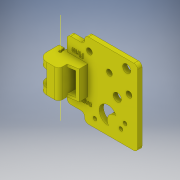
# Autodesk Inventor part: Catch
Saved by Autodesk Inventor 2016 (Build 200138000, 138)
## iProperties
Created: 2016-11-16
Part Number: Catch
Material: ABS Plastic
Document SubType Name: Modeling
Designer: brownadam
Density: 1.06 g/cm^3
Appearance: Yellow
Author: brownadam
Autodesk Inventor part; units mm, degrees
note: some values were not read from the file. Chosen so that the rebuilt part matches the saved one: direction of "Emboss1".
ref_plane "YZ Plane" through (0, 0, 0) normal (1, 0, 0) x (0, 1, 0)
ref_plane "XZ Plane" through (0, 0, 0) normal (0, 1, 0) x (-1, 0, 0)
ref_plane "XY Plane" through (0, 0, 0) normal (0, 0, 1) x (1, 0, 0)
sketch "Sketch1" plane through (0, 0, 0) normal (0, 0, 1) x (1, 0, 0)
  line L0 (30.48, 0) -> (30.48, 14.732)
  line L1 (28.8925, 16.3195) -> (9.2075, 16.3195)
  line L2 (0, 11.176) -> (0, 3.429)
  line L3 (7.62, 14.732) -> (7.62, 14.351)
  line L4 (6.0325, 12.7635) -> (1.5875, 12.7635)
  line L5 (7.62, 0) -> (30.48, 0) construction
  arc A0 (1.5875, 12.7635) -> (0, 11.176) centre (1.5875, 11.176) ccw
  arc A1 (6.0325, 12.7635) -> (7.62, 14.351) centre (6.0325, 14.351) ccw
  arc A2 (9.2075, 16.3195) -> (7.62, 14.732) centre (9.2075, 14.732) ccw
  arc A3 (30.48, 14.732) -> (28.8925, 16.3195) centre (28.8925, 14.732) ccw
  line L6 (0, 3.429) -> (2.2606, 3.429)
  line L7 (2.2606, 3.429) -> (2.2606, 0)
  line L8 (30.48, 0) -> (2.2606, 0) construction
  line L9 (30.48, 0) -> (30.48, -14.732)
  line L10 (28.8925, -16.3195) -> (9.2075, -16.3195)
  line L11 (0, -11.176) -> (0, -3.429)
  line L12 (6.0325, -12.7635) -> (1.5875, -12.7635)
  arc A4 (0, -11.176) -> (1.5875, -12.7635) centre (1.5875, -11.176) ccw
  arc A5 (7.62, -14.351) -> (6.0325, -12.7635) centre (6.0325, -14.351) ccw
  arc A6 (7.62, -14.732) -> (9.2075, -16.3195) centre (9.2075, -14.732) ccw
  arc A7 (28.8925, -16.3195) -> (30.48, -14.732) centre (28.8925, -14.732) ccw
  line L13 (0, -3.429) -> (2.2606, -3.429)
  line L14 (2.2606, -3.429) -> (2.2606, 0)
  line L15 (7.62, -14.732) -> (7.62, -14.351)
  point P0 (0, 0)
  dimension "d4" = 30.48
  dimension "d5" = 7.62
  dimension "d6" = 3.556
  dimension "d8" = 1.5875
  dimension "d9" = 1.5875
  dimension "d10" = 1.5875
  dimension "d11" = 1.5875
  dimension "d13" = 16.3195
  dimension "d14" = 2.2606
  dimension "d16" = 3.429
  constraints: 32 end point, 16 point on circle, 14 symmetric about line, 8 centre point, 8 tangent, 2 horizontal alignment, 2 perpendicular, 1 collinear, 1 horizontal, 1 parallel, 1 point on line, 1 vertical, 1 vertical alignment, 4 other
  measures "d4" distance between parallel lines of L0 L2
  measures "d5" distance between parallel lines of L3 L2
  measures "d6" distance between parallel lines of L4 L1
  measures "d8" radius of A0
  measures "d9" radius of A1
  measures "d10" radius of A2
  measures "d11" radius of A3
  measures "d13" distance between parallel lines of L5 L1
  measures "d14" distance of L2.end L6.end
  measures "d16" distance from line of L7.end L6
extrude "Extrusion1" add sketch "Sketch1" against normal blind 1.905
sketch "Sketch2" plane through (0, 0, 0) normal (0, 0, 1) x (1, 0, 0)
  line L0 (30.48, 14.732) -> (30.48, -14.732) projected
  line L1 (9.2075, 16.3195) -> (28.8925, 16.3195) projected
  line L2 (-4.318, 6.1595) -> (9.017, 6.1595)
  line L3 (9.017, 6.1595) -> (9.017, -6.1595)
  line L4 (9.017, -6.1595) -> (-4.318, -6.1595)
  line L5 (-4.318, -6.1595) -> (-4.318, 6.1595)
  point P0 (0, 0)
  dimension "d19" = 13.335
  dimension "d20" = 12.319
  dimension "d21" = 10.16
  dimension "d22" = 21.463
  constraints: 8 end point, 2 parallel, 1 horizontal, 1 perpendicular
  measures "d19" distance of L2.start L2.end
  measures "d20" distance of L2.end L3.end
  measures "d21" distance between parallel lines of L1 L2
  measures "d22" distance between parallel lines of L0 L3
extrude "Extrusion2" add sketch "Sketch2" along normal blind 8.255
sketch "Sketch3" plane through (0, 0, 8.255) normal (0, 0, 1) x (1, 0, 0)
  line L0 (9.017, 6.1595) -> (-4.318, 6.1595) projected
  line L1 (-4.318, 6.1595) -> (-4.318, -6.1595) projected
  line L2 (-4.318, -6.1595) -> (9.017, -6.1595) projected
  line L3 (9.017, -6.1595) -> (9.017, 6.1595) projected
  line L4 (-4.318, 3.429) -> (-0.508, 3.429)
  line L5 (-0.508, 3.429) -> (-0.508, -3.429)
  line L6 (-0.508, -3.429) -> (-4.318, -3.429)
  line L7 (-4.318, -3.429) -> (-4.318, 3.429)
  line L8 (9.017, 5.0165) -> (4.572, 5.0165)
  line L9 (4.572, 5.0165) -> (4.572, -5.0165)
  line L10 (4.572, -5.0165) -> (9.017, -5.0165)
  line L11 (9.017, -5.0165) -> (9.017, 5.0165)
  line L12 (4.572, 5.0165) -> (7.747, 5.0165)
  line L13 (7.747, 5.0165) -> (7.747, -5.0165)
  line L14 (7.747, -5.0165) -> (4.572, -5.0165)
  line L15 (4.572, -5.0165) -> (4.572, 5.0165)
  line L16 (4.572, 5.0165) -> (4.572, 6.1595)
  line L17 (4.572, -5.0165) -> (4.572, -6.1595)
  point P0 (0, 0)
  dimension "d25" = 3.81
  dimension "d27" = 2.7305
  dimension "d28" = 5.08
  dimension "d29" = 1.143
  dimension "d30" = 1.143
  dimension "d31" = 1.27
  dimension "d38" = 2.7305
  constraints: 28 end point, 6 parallel, 6 point on line, 4 perpendicular, 3 horizontal
  measures "d25" distance of L5.end L6.end
  measures "d27" distance between parallel lines of L0 L4
  measures "d28" distance between parallel lines of L9 L5
  measures "d29" distance between parallel lines of L2 L10
  measures "d30" distance between parallel lines of L0 L8
  measures "d31" distance between parallel lines of L13 L11
  measures "d38" distance between parallel lines of L6 L2
extrude "Extrusion3" cut sketch "Sketch3" against normal through all contours L4 L5 L6 L1
extrude "Extrusion4" cut sketch "Sketch3" against normal up to surface (8.255 mm away) contours L8 L13 L10 L9
sketch "Sketch4" plane through (0, 0, 0) normal (0, 0, -1) x (-1, 0, 0)
  line L0 (0.508, 3.429) -> (0, 3.429)
  line L1 (0, 3.429) -> (0, 6.1595)
  line L2 (0, 6.1595) -> (0.508, 6.1595)
  line L3 (0.508, 6.1595) -> (0.508, 3.429)
  line L4 (0.508, -3.429) -> (0, -3.429)
  line L5 (0, -3.429) -> (0, -6.1595)
  line L6 (0, -6.1595) -> (0.508, -6.1595)
  line L7 (0.508, -6.1595) -> (0.508, -3.429)
  line L8 (4.318, -3.429) -> (0.508, -3.429) projected
  line L9 (0.508, -3.429) -> (0.508, 3.429) projected
  line L10 (0.508, 3.429) -> (4.318, 3.429) projected
  line L11 (4.318, 3.429) -> (4.318, 6.1595) projected
  line L12 (4.318, 6.1595) -> (0, 6.1595) projected
  line L13 (0, 3.429) -> (0, 6.1595) projected
  line L14 (-2.2606, 3.429) -> (0, 3.429) projected
  line L15 (-2.2606, -3.429) -> (-2.2606, 3.429) projected
  line L16 (0, -3.429) -> (-2.2606, -3.429) projected
  line L17 (0, -6.1595) -> (0, -3.429) projected
  line L18 (0, -6.1595) -> (4.318, -6.1595) projected
  line L19 (4.318, -6.1595) -> (4.318, -3.429) projected
  line L20 (4.318, 6.1595) -> (0.508, 6.1595)
  line L21 (0.508, 6.1595) -> (0.508, 3.429)
  line L22 (0.508, 3.429) -> (4.318, 3.429)
  line L23 (4.318, 3.429) -> (4.318, 6.1595)
  line L24 (0.508, -3.429) -> (4.318, -3.429) projected
  line L25 (4.318, -3.429) -> (0.508, -3.429)
  line L26 (0.508, -3.429) -> (0.508, -6.1595)
  line L27 (0.508, -6.1595) -> (4.318, -6.1595)
  line L28 (4.318, -6.1595) -> (4.318, -3.429)
  point P0 (0, 0)
  constraints: 32 end point, 8 parallel, 4 horizontal, 4 perpendicular
extrude "Extrusion5" add sketch "Sketch4" along normal up to surface (1.905 mm away) contours L0 L1 L2 L3 | L7 L6 L5 L4
extrude "Extrusion6" add sketch "Sketch4" along normal blind 0.889 contours L3 L12 L11 L10 | L8 L19 L18 L7
sketch "Sketch6" plane through (0, -6.1595, 0) normal (0, -1, 0) x (1, 0, 0)
  line L0 (-4.318, 8.255) -> (9.017, 8.255) projected
  line L1 (-4.318, 8.255) -> (-4.318, -0.889) projected
  line L2 (-0.508, -0.889) -> (-4.318, -0.889) projected
  line L3 (9.017, 0) -> (9.017, 3.81)
  line L4 (9.017, 0) -> (9.017, 8.255) projected
  line L5 (7.747, 8.255) -> (4.572, 8.255) construction
  line L6 (4.572, 8.255) -> (4.572, 0) construction
  line L7 (4.572, 8.255) -> (4.572, 0) construction
  line L8 (9.017, 3.81) -> (4.572, 4.572)
  line L9 (4.572, 8.255) -> (4.572, 0) projected
  line L10 (4.572, 4.572) -> (4.572, 8.255)
  line L11 (4.572, 8.255) -> (-4.318, 8.255)
  line L12 (-4.318, -0.889) -> (-4.318, 8.255) projected
  line L13 (-4.318, 8.255) -> (-4.318, -0.889)
  line L14 (-4.318, -0.889) -> (-2.032, -0.889)
  line L15 (-2.032, -0.889) -> (-1.905, 0.8471)
  line L16 (-0.508, -0.889) -> (-0.508, -1.905) projected
  line L17 (-0.508, -0.889) -> (-1.143, -0.889)
  line L18 (-1.143, -0.889) -> (-1.27, 0.8471)
  line L19 (-1.905, 0.8471) -> (-1.27, 0.8471) construction
  arc A0 (-1.27, 0.8471) -> (-1.905, 0.8471) centre (-1.5875, 1.3284) ccw
  line L20 (4.572, 8.255) -> (9.017, 8.255)
  line L21 (9.017, 8.255) -> (9.017, 3.81)
  point P0 (-1.5875, 0.8471)
  point P1 (-1.5875, 1.905)
  dimension "d41" = 3.81
  dimension "d42" = 3.683
  dimension "d43" = 2.286
  dimension "d44" = 0.635
  dimension "d45" = 1.1532
  dimension "d46" = 0.635
  dimension "d47" = 6.35
  dimension "d48" = 1.7361
  constraints: 26 end point, 5 collinear, 4 point on line, 3 point on circle, 2 horizontal, 1 centre point, 1 coincident, 1 equal length, 1 midpoint, 1 vertical alignment
  measures "d41" distance of L3.start L3.end
  measures "d42" distance of L5.end L8.end
  measures "d43" distance of L1.end L14.end
  measures "d44" distance of L2.start L17.end
  measures "d45" diameter of A0
  measures "d46" distance of L18.end L15.end
  measures "d47" distance from line of point (-1.588, 1.905) L11
  measures "d48" vertical distance of L14.end L15.end
extrude "Extrusion7" cut sketch "Sketch6" against normal through all
fillet "Fillet1" radius 1.5875 1 edges at (4.572, 0, 8.255)
fillet "Fillet2" radius 3.81 2 edges at (-4.318, -4.7942, 8.255) (-4.318, 4.7943, 8.255)
sketch "Sketch7" plane through (0, 0, 0) normal (0, 0, 1) x (1, 0, 0)
  arc A0 (21.1133, -7.0794) -> (17.8739, -12.4712) centre (17.6502, -8.6677) ccw
  arc A1 (21.1133, -7.0794) -> (17.8739, -12.4712) centre (20.916, -10.6299) ccw
  line L0 (7.3431, 7.1617) -> (-0.2045, 7.1617) construction
  line L1 (-0.2045, 7.1617) -> (-0.2045, 10.7769) construction
  line L2 (-0.2045, 10.7769) -> (7.3431, 10.7769) construction
  line L3 (7.3431, 10.7769) -> (7.3431, 7.1617) construction
  line L4 (0.5888, -7.1353) -> (10.8131, -7.1353) construction
  line L5 (10.8131, -7.1353) -> (10.8131, -9.1082) construction
  line L6 (10.8131, -9.1082) -> (0.5888, -9.1082) construction
  line L7 (0.5888, -9.1082) -> (0.5888, -7.1353) construction
  spline S0 degree 2 poles (1.3128, -9.1082) (1.106, -9.1082) (0.8157, -9.0218) (0.6876, -8.96) knots 0 0 0 1 2 2 2
  line L8 (0.6876, -8.96) -> (0.6876, -8.642)
  line L9 (0.6876, -8.642) -> (0.7061, -8.642)
  spline S1 degree 2 poles (0.7061, -8.642) (0.8312, -8.7594) (1.1477, -8.889) (1.2943, -8.889) knots 0 0 0 1 2 2 2
  spline S2 degree 2 poles (1.2943, -8.889) (1.5043, -8.889) (1.7188, -8.7146) (1.7188, -8.571) knots 0 0 0 1 2 2 2
  spline S3 degree 2 poles (1.7188, -8.571) (1.7188, -8.4568) (1.6062, -8.3148) (1.4842, -8.2792) knots 0 0 0 1 2 2 2
  spline S4 degree 2 poles (1.4842, -8.2792) (1.3962, -8.2545) (1.2495, -8.2206) (1.1399, -8.1928) knots 0 0 0 1 2 2 2
  spline S5 degree 2 poles (1.1399, -8.1928) (1.0411, -8.1665) (0.8852, -8.0878) (0.825, -8.0245) knots 0 0 0 1 2 2 2
  spline S6 degree 2 poles (0.825, -8.0245) (0.7663, -7.9612) (0.7015, -7.7914) (0.7015, -7.6803) knots 0 0 0 1 2 2 2
  spline S7 degree 2 poles (0.7015, -7.6803) (0.7015, -7.4487) (1.0627, -7.1353) (1.3422, -7.1353) knots 0 0 0 1 2 2 2
  spline S8 degree 2 poles (1.3422, -7.1353) (1.5027, -7.1353) (1.7868, -7.1986) (1.9087, -7.2588) knots 0 0 0 1 2 2 2
  line L10 (1.9087, -7.2588) -> (1.9087, -7.5614)
  line L11 (1.9087, -7.5614) -> (1.8902, -7.5614)
  spline S9 degree 2 poles (1.8902, -7.5614) (1.7991, -7.478) (1.5151, -7.3545) (1.3591, -7.3545) knots 0 0 0 1 2 2 2
  spline S10 degree 2 poles (1.3591, -7.3545) (1.1832, -7.3545) (0.9655, -7.5197) (0.9655, -7.654) knots 0 0 0 1 2 2 2
  spline S11 degree 2 poles (0.9655, -7.654) (0.9655, -7.7744) (1.0936, -7.918) (1.214, -7.9504) knots 0 0 0 1 2 2 2
  spline S12 degree 2 poles (1.214, -7.9504) (1.2943, -7.972) (1.5274, -8.0276) (1.6046, -8.0508) knots 0 0 0 1 2 2 2
  spline S13 degree 2 poles (1.6046, -8.0508) (1.8007, -8.111) (1.9828, -8.3533) (1.9828, -8.5309) knots 0 0 0 1 2 2 2
  spline S14 degree 2 poles (1.9828, -8.5309) (1.9828, -8.6436) (1.8917, -8.8597) (1.8099, -8.9353) knots 0 0 0 1 2 2 2
  spline S15 degree 2 poles (1.8099, -8.9353) (1.7188, -9.0187) (1.4873, -9.1082) (1.3128, -9.1082) knots 0 0 0 1 2 2 2
  spline S16 degree 2 poles (2.8427, -9.1067) (2.5, -9.1067) (2.1233, -8.7223) (2.1233, -8.3672) knots 0 0 0 1 2 2 2
  spline S17 degree 2 poles (2.1233, -8.3672) (2.1233, -8.0183) (2.4892, -7.6046) (2.784, -7.6046) knots 0 0 0 1 2 2 2
  spline S18 degree 2 poles (2.784, -7.6046) (2.9168, -7.6046) (3.1221, -7.6818) (3.1978, -7.7636) knots 0 0 0 1 2 2 2
  spline S19 degree 2 poles (3.1978, -7.7636) (3.275, -7.8454) (3.3568, -8.0816) (3.3568, -8.253) knots 0 0 0 1 2 2 2
  line L12 (3.3568, -8.253) -> (3.3568, -8.3842)
  line L13 (3.3568, -8.3842) -> (2.3672, -8.3842)
  spline S20 degree 2 poles (2.3672, -8.3842) (2.3672, -8.6328) (2.6173, -8.8967) (2.8396, -8.8967) knots 0 0 0 1 2 2 2
  spline S21 degree 2 poles (2.8396, -8.8967) (2.9183, -8.8967) (3.0712, -8.8612) (3.1329, -8.8335) knots 0 0 0 1 2 2 2
  spline S22 degree 2 poles (3.1329, -8.8335) (3.1978, -8.8026) (3.2873, -8.7485) (3.3166, -8.7238) knots 0 0 0 1 2 2 2
  line L14 (3.3166, -8.7238) -> (3.3305, -8.7238)
  line L15 (3.3305, -8.7238) -> (3.3305, -8.9863)
  spline S23 degree 2 poles (3.3305, -8.9863) (3.2888, -9.0033) (3.1623, -9.0527) (3.1129, -9.0666) knots 0 0 0 1 2 2 2
  spline S24 degree 2 poles (3.1129, -9.0666) (3.0434, -9.0866) (2.9292, -9.1067) (2.8427, -9.1067) knots 0 0 0 1 2 2 2
  spline S25 degree 2 poles (3.1221, -8.2005) (3.119, -8.1033) (3.0789, -7.9612) (3.0403, -7.9134) knots 0 0 0 1 2 2 2
  spline S26 degree 2 poles (3.0403, -7.9134) (2.9986, -7.8593) (2.8674, -7.8022) (2.7701, -7.8022) knots 0 0 0 1 2 2 2
  spline S27 degree 2 poles (2.7701, -7.8022) (2.6744, -7.8022) (2.5401, -7.8593) (2.4846, -7.9149) knots 0 0 0 1 2 2 2
  spline S28 degree 2 poles (2.4846, -7.9149) (2.4305, -7.972) (2.3749, -8.1094) (2.3672, -8.2005) knots 0 0 0 1 2 2 2
  line L16 (2.3672, -8.2005) -> (3.1221, -8.2005)
  line L17 (4.723, -9.0743) -> (4.4822, -9.0743)
  line L18 (4.4822, -9.0743) -> (4.4822, -8.2592)
  spline S29 degree 2 poles (4.4822, -8.2592) (4.4822, -8.1604) (4.4637, -7.9906) (4.4359, -7.9396) knots 0 0 0 1 2 2 2
  spline S30 degree 2 poles (4.4359, -7.9396) (4.4065, -7.8856) (4.3016, -7.8331) (4.212, -7.8331) knots 0 0 0 1 2 2 2
  spline S31 degree 2 poles (4.212, -7.8331) (4.1225, -7.8331) (3.9326, -7.9288) (3.8415, -8.006) knots 0 0 0 1 2 2 2
  line L19 (3.8415, -8.006) -> (3.8415, -9.0743)
  line L20 (3.8415, -9.0743) -> (3.6007, -9.0743)
  line L21 (3.6007, -9.0743) -> (3.6007, -7.6448)
  line L22 (3.6007, -7.6448) -> (3.8415, -7.6448)
  line L23 (3.8415, -7.6448) -> (3.8415, -7.8038)
  spline S32 degree 2 poles (3.8415, -7.8038) (3.9496, -7.7065) (4.158, -7.6046) (4.2753, -7.6046) knots 0 0 0 1 2 2 2
  spline S33 degree 2 poles (4.2753, -7.6046) (4.4853, -7.6046) (4.723, -7.8825) (4.723, -8.1465) knots 0 0 0 1 2 2 2
  line L24 (4.723, -8.1465) -> (4.723, -9.0743)
  spline S34 degree 2 poles (5.447, -9.1082) (5.3035, -9.1082) (5.0549, -9.0311) (4.9731, -8.9878) knots 0 0 0 1 2 2 2
  line L25 (4.9731, -8.9878) -> (4.9731, -8.7177)
  line L26 (4.9731, -8.7177) -> (4.9854, -8.7177)
  spline S35 degree 2 poles (4.9854, -8.7177) (5.0163, -8.7424) (5.0997, -8.801) (5.1691, -8.8335) knots 0 0 0 1 2 2 2
  spline S36 degree 2 poles (5.1691, -8.8335) (5.2294, -8.8628) (5.3776, -8.906) (5.4563, -8.906) knots 0 0 0 1 2 2 2
  spline S37 degree 2 poles (5.4563, -8.906) (5.5134, -8.906) (5.6446, -8.8798) (5.6755, -8.8582) knots 0 0 0 1 2 2 2
  spline S38 degree 2 poles (5.6755, -8.8582) (5.7203, -8.8288) (5.7604, -8.7624) (5.7604, -8.6945) knots 0 0 0 1 2 2 2
  spline S39 degree 2 poles (5.7604, -8.6945) (5.7604, -8.6096) (5.6678, -8.5216) (5.5489, -8.4923) knots 0 0 0 1 2 2 2
  spline S40 degree 2 poles (5.5489, -8.4923) (5.5026, -8.4815) (5.3544, -8.4506) (5.2911, -8.4336) knots 0 0 0 1 2 2 2
  spline S41 degree 2 poles (5.2911, -8.4336) (5.1275, -8.3858) (4.9793, -8.1882) (4.9793, -8.0477) knots 0 0 0 1 2 2 2
  spline S42 degree 2 poles (4.9793, -8.0477) (4.9793, -7.8532) (5.271, -7.6108) (5.5119, -7.6108) knots 0 0 0 1 2 2 2
  spline S43 degree 2 poles (5.5119, -7.6108) (5.6307, -7.6108) (5.8716, -7.6695) (5.9534, -7.7142) knots 0 0 0 1 2 2 2
  line L27 (5.9534, -7.7142) -> (5.9534, -7.972)
  line L28 (5.9534, -7.972) -> (5.941, -7.972)
  spline S44 degree 2 poles (5.941, -7.972) (5.8484, -7.8979) (5.623, -7.813) (5.5072, -7.813) knots 0 0 0 1 2 2 2
  spline S45 degree 2 poles (5.5072, -7.813) (5.3884, -7.813) (5.2247, -7.9134) (5.2247, -8.0137) knots 0 0 0 1 2 2 2
  spline S46 degree 2 poles (5.2247, -8.0137) (5.2247, -8.1048) (5.322, -8.1928) (5.43, -8.2206) knots 0 0 0 1 2 2 2
  spline S47 degree 2 poles (5.43, -8.2206) (5.4825, -8.2345) (5.6153, -8.2623) (5.6879, -8.2792) knots 0 0 0 1 2 2 2
  spline S48 degree 2 poles (5.6879, -8.2792) (5.8453, -8.3194) (6.0059, -8.5031) (6.0059, -8.6621) knots 0 0 0 1 2 2 2
  spline S49 degree 2 poles (6.0059, -8.6621) (6.0059, -8.7547) (5.9333, -8.9184) (5.8623, -8.9786) knots 0 0 0 1 2 2 2
  spline S50 degree 2 poles (5.8623, -8.9786) (5.7867, -9.0419) (5.5937, -9.1082) (5.447, -9.1082) knots 0 0 0 1 2 2 2
  line L29 (6.4752, -9.0743) -> (6.2343, -9.0743)
  line L30 (6.2343, -9.0743) -> (6.2343, -7.6448)
  line L31 (6.2343, -7.6448) -> (6.4752, -7.6448)
  line L32 (6.4752, -7.6448) -> (6.4752, -9.0743)
  line L33 (6.4922, -7.407) -> (6.2189, -7.407)
  line L34 (6.2189, -7.407) -> (6.2189, -7.1569)
  line L35 (6.2189, -7.1569) -> (6.4922, -7.1569)
  line L36 (6.4922, -7.1569) -> (6.4922, -7.407)
  spline S51 degree 2 poles (7.2609, -9.1021) (7.0649, -9.1021) (6.8441, -8.8782) (6.8441, -8.6359) knots 0 0 0 1 2 2 2
  line L37 (6.8441, -8.6359) -> (6.8441, -7.8439)
  line L38 (6.8441, -7.8439) -> (6.682, -7.8439)
  line L39 (6.682, -7.8439) -> (6.682, -7.6448)
  line L40 (6.682, -7.6448) -> (6.8441, -7.6448)
  line L41 (6.8441, -7.6448) -> (6.8441, -7.2341)
  line L42 (6.8441, -7.2341) -> (7.085, -7.2341)
  line L43 (7.085, -7.2341) -> (7.085, -7.6448)
  line L44 (7.085, -7.6448) -> (7.528, -7.6448)
  line L45 (7.528, -7.6448) -> (7.528, -7.8439)
  line L46 (7.528, -7.8439) -> (7.085, -7.8439)
  line L47 (7.085, -7.8439) -> (7.085, -8.5247)
  spline S52 degree 2 poles (7.085, -8.5247) (7.085, -8.6328) (7.0927, -8.7516) (7.1189, -8.8026) knots 0 0 0 1 2 2 2
  spline S53 degree 2 poles (7.1189, -8.8026) (7.1405, -8.8473) (7.2378, -8.8921) (7.3212, -8.8921) knots 0 0 0 1 2 2 2
  spline S54 degree 2 poles (7.3212, -8.8921) (7.3798, -8.8921) (7.4894, -8.8566) (7.5141, -8.8458) knots 0 0 0 1 2 2 2
  line L48 (7.5141, -8.8458) -> (7.528, -8.8458)
  line L49 (7.528, -8.8458) -> (7.528, -9.0619)
  spline S55 degree 2 poles (7.528, -9.0619) (7.4601, -9.0805) (7.3212, -9.1021) (7.2609, -9.1021) knots 0 0 0 1 2 2 2
  line L50 (7.951, -9.0743) -> (7.7102, -9.0743)
  line L51 (7.7102, -9.0743) -> (7.7102, -7.6448)
  line L52 (7.7102, -7.6448) -> (7.951, -7.6448)
  line L53 (7.951, -7.6448) -> (7.951, -9.0743)
  line L54 (7.968, -7.407) -> (7.6947, -7.407)
  line L55 (7.6947, -7.407) -> (7.6947, -7.1569)
  line L56 (7.6947, -7.1569) -> (7.968, -7.1569)
  line L57 (7.968, -7.1569) -> (7.968, -7.407)
  line L58 (9.4268, -7.6448) -> (8.8881, -9.0743)
  line L59 (8.8881, -9.0743) -> (8.6719, -9.0743)
  line L60 (8.6719, -9.0743) -> (8.1378, -7.6448)
  line L61 (8.1378, -7.6448) -> (8.3987, -7.6448)
  line L62 (8.3987, -7.6448) -> (8.7893, -8.7455)
  line L63 (8.7893, -8.7455) -> (9.1768, -7.6448)
  line L64 (9.1768, -7.6448) -> (9.4268, -7.6448)
  spline S56 degree 2 poles (10.2296, -9.1067) (9.8869, -9.1067) (9.5102, -8.7223) (9.5102, -8.3672) knots 0 0 0 1 2 2 2
  spline S57 degree 2 poles (9.5102, -8.3672) (9.5102, -8.0183) (9.8761, -7.6046) (10.1709, -7.6046) knots 0 0 0 1 2 2 2
  spline S58 degree 2 poles (10.1709, -7.6046) (10.3037, -7.6046) (10.509, -7.6818) (10.5847, -7.7636) knots 0 0 0 1 2 2 2
  spline S59 degree 2 poles (10.5847, -7.7636) (10.6618, -7.8454) (10.7437, -8.0816) (10.7437, -8.253) knots 0 0 0 1 2 2 2
  line L65 (10.7437, -8.253) -> (10.7437, -8.3842)
  line L66 (10.7437, -8.3842) -> (9.7541, -8.3842)
  spline S60 degree 2 poles (9.7541, -8.3842) (9.7541, -8.6328) (10.0042, -8.8967) (10.2265, -8.8967) knots 0 0 0 1 2 2 2
  spline S61 degree 2 poles (10.2265, -8.8967) (10.3052, -8.8967) (10.4581, -8.8612) (10.5198, -8.8335) knots 0 0 0 1 2 2 2
  spline S62 degree 2 poles (10.5198, -8.8335) (10.5847, -8.8026) (10.6742, -8.7485) (10.7035, -8.7238) knots 0 0 0 1 2 2 2
  line L67 (10.7035, -8.7238) -> (10.7174, -8.7238)
  line L68 (10.7174, -8.7238) -> (10.7174, -8.9863)
  spline S63 degree 2 poles (10.7174, -8.9863) (10.6757, -9.0033) (10.5492, -9.0527) (10.4998, -9.0666) knots 0 0 0 1 2 2 2
  spline S64 degree 2 poles (10.4998, -9.0666) (10.4303, -9.0866) (10.316, -9.1067) (10.2296, -9.1067) knots 0 0 0 1 2 2 2
  spline S65 degree 2 poles (10.509, -8.2005) (10.5059, -8.1033) (10.4658, -7.9612) (10.4272, -7.9134) knots 0 0 0 1 2 2 2
  spline S66 degree 2 poles (10.4272, -7.9134) (10.3855, -7.8593) (10.2543, -7.8022) (10.157, -7.8022) knots 0 0 0 1 2 2 2
  spline S67 degree 2 poles (10.157, -7.8022) (10.0613, -7.8022) (9.927, -7.8593) (9.8714, -7.9149) knots 0 0 0 1 2 2 2
  spline S68 degree 2 poles (9.8714, -7.9149) (9.8174, -7.972) (9.7618, -8.1094) (9.7541, -8.2005) knots 0 0 0 1 2 2 2
  line L69 (9.7541, -8.2005) -> (10.509, -8.2005)
  line L70 (6.0108, 7.3994) -> (6.8969, 7.3994)
  line L71 (6.8969, 7.3994) -> (6.8969, 7.9367)
  line L72 (6.8969, 7.9367) -> (6.0479, 7.9367)
  line L73 (6.0479, 7.9367) -> (6.0479, 8.1621)
  line L74 (6.0479, 8.1621) -> (6.8969, 8.1621)
  line L75 (6.8969, 8.1621) -> (6.8969, 9.0791)
  line L76 (6.8969, 9.0791) -> (7.1501, 9.0791)
  line L77 (7.1501, 9.0791) -> (7.1501, 7.1741)
  line L78 (7.1501, 7.1741) -> (6.0108, 7.1741)
  line L79 (6.0108, 7.1741) -> (6.0108, 7.3994)
  line L80 (5.5569, 9.0791) -> (5.7978, 9.0791)
  line L81 (5.7978, 9.0791) -> (5.7978, 7.6495)
  line L82 (5.7978, 7.6495) -> (5.5569, 7.6495)
  line L83 (5.5569, 7.6495) -> (5.5569, 9.0791)
  line L84 (5.54, 7.4118) -> (5.8132, 7.4118)
  line L85 (5.8132, 7.4118) -> (5.8132, 7.1617)
  line L86 (5.8132, 7.1617) -> (5.54, 7.1617)
  line L87 (5.54, 7.1617) -> (5.54, 7.4118)
  line L88 (4.4454, 7.9073) -> (4.4578, 7.9073)
  spline S69 degree 2 poles (4.4578, 7.9073) (4.4856, 7.8996) (4.5458, 7.8965) (4.5875, 7.8965) knots 0 0 0 1 2 2 2
  spline S70 degree 2 poles (4.5875, 7.8965) (4.6847, 7.8965) (4.8761, 7.9814) (4.9626, 8.0648) knots 0 0 0 1 2 2 2
  line L89 (4.9626, 8.0648) -> (4.9626, 9.0791)
  line L90 (4.9626, 9.0791) -> (5.2034, 9.0791)
  line L91 (5.2034, 9.0791) -> (5.2034, 7.6495)
  line L92 (5.2034, 7.6495) -> (4.9626, 7.6495)
  line L93 (4.9626, 7.6495) -> (4.9626, 7.8626)
  spline S71 degree 2 poles (4.9626, 7.8626) (4.8314, 7.7452) (4.6353, 7.6495) (4.5427, 7.6495) knots 0 0 0 1 2 2 2
  spline S72 degree 2 poles (4.5427, 7.6495) (4.5056, 7.6495) (4.4686, 7.6526) (4.4454, 7.6572) knots 0 0 0 1 2 2 2
  line L94 (4.4454, 7.6572) -> (4.4454, 7.9073)
  line L95 (2.6377, 9.0791) -> (2.6377, 8.2516)
  spline S73 degree 2 poles (2.6377, 8.2516) (2.6377, 8.1528) (2.6531, 7.9845) (2.6778, 7.9382) knots 0 0 0 1 2 2 2
  spline S74 degree 2 poles (2.6778, 7.9382) (2.7025, 7.8873) (2.7967, 7.8379) (2.8785, 7.8379) knots 0 0 0 1 2 2 2
  spline S75 degree 2 poles (2.8785, 7.8379) (2.9526, 7.8379) (3.1224, 7.929) (3.212, 8.0154) knots 0 0 0 1 2 2 2
  spline S76 degree 2 poles (3.212, 8.0154) (3.2104, 8.037) (3.2073, 8.0972) (3.2073, 8.1374) knots 0 0 0 1 2 2 2
  line L96 (3.2073, 8.1374) -> (3.2073, 9.0791)
  line L97 (3.2073, 9.0791) -> (3.4482, 9.0791)
  line L98 (3.4482, 9.0791) -> (3.4482, 8.2516)
  spline S77 degree 2 poles (3.4482, 8.2516) (3.4482, 8.1528) (3.4636, 7.9845) (3.4883, 7.9382) knots 0 0 0 1 2 2 2
  spline S78 degree 2 poles (3.4883, 7.9382) (3.513, 7.8873) (3.6072, 7.8379) (3.689, 7.8379) knots 0 0 0 1 2 2 2
  spline S79 degree 2 poles (3.689, 7.8379) (3.7662, 7.8379) (3.9375, 7.9351) (4.0178, 8.0108) knots 0 0 0 1 2 2 2
  line L99 (4.0178, 8.0108) -> (4.0178, 9.0791)
  line L100 (4.0178, 9.0791) -> (4.2586, 9.0791)
  line L101 (4.2586, 9.0791) -> (4.2586, 7.6495)
  line L102 (4.2586, 7.6495) -> (4.0178, 7.6495)
  line L103 (4.0178, 7.6495) -> (4.0178, 7.807)
  spline S80 degree 2 poles (4.0178, 7.807) (3.9236, 7.7128) (3.7384, 7.6094) (3.6272, 7.6094) knots 0 0 0 1 2 2 2
  spline S81 degree 2 poles (3.6272, 7.6094) (3.5006, 7.6094) (3.3046, 7.7252) (3.2536, 7.8564) knots 0 0 0 1 2 2 2
  spline S82 degree 2 poles (3.2536, 7.8564) (3.144, 7.7344) (2.9372, 7.6094) (2.8168, 7.6094) knots 0 0 0 1 2 2 2
  spline S83 degree 2 poles (2.8168, 7.6094) (2.7241, 7.6094) (2.5728, 7.6665) (2.5173, 7.7313) knots 0 0 0 1 2 2 2
  spline S84 degree 2 poles (2.5173, 7.7313) (2.4602, 7.7962) (2.3969, 7.9907) (2.3969, 8.1374) knots 0 0 0 1 2 2 2
  line L104 (2.3969, 8.1374) -> (2.3969, 9.0791)
  line L105 (2.3969, 9.0791) -> (2.6377, 9.0791)
  point P0 (0, 0)
  point P1 (9.6586, 11.176)
  point P2 (18.2844, 7.5159)
  point P3 (25.7686, 12.7635)
  point P4 (26.7834, 3.5835)
  point P5 (21.7094, 0)
  point P6 (25.0709, -8.0867)
  point P7 (23.295, -11.0042)
  point P8 (12.0687, -12.7635)
  dimension "d53" = 7.62
  dimension "d54" = 7.112
  constraints: 5 point on circle, 2 centre point, 1 coincident, 4 other
  measures "d53" diameter of A0
  measures "d54" diameter of A1
extrude "Extrusion8" cut sketch "Sketch7" against normal through all contours A1 A0
hole "Hole1" at (25.0709, -8.0867, 0) at (12.0687, -12.7635, 0) at (23.295, -11.0042, 0) direction (0, 0, -1) diameter 1.651 end through all
hole "Hole2" at (9.6586, 11.176, 0) at (18.2844, 7.5159, 0) at (26.7834, 3.5835, 0) direction (0, 0, -1) diameter 2.54 end through all
hole "Hole3" at (25.7686, 12.7635, 0) at (21.7094, 0, 0) direction (0, 0, -1) diameter 3.556 end through all
emboss "Emboss1" sketch "Sketch7" operation add depth 0.3175 direction (0, 0, -1) contours S0 L8 L9 S1 S2 S3 S4 S5 S6 S7 S8 L10 L11 S9 S10 S11 S12 S13 S14 S15 | S16 S17 S18 S19 L12 L13 S20 S21 S22 L14 L15 S23 S24 | L17 L18 S29 S30 S31 L19 L20 L21 L22 L23 S32 S33 L24 | S34 L25 L26 S35 S36 S37 S38 S39 S40 S41 S42 S43 L27 L28 S44 S45 S46 S47 S48 S49 S50 | L29 L30 L31 L32 | L33 L34 L35 L36 | S51 L37 L38 L39 L40 L41 L42 L43 L44 L45 L46 L47 S52 S53 S54 L48 L49 S55 | L50 L51 L52 L53 | L54 L55 L56 L57 | L58 L59 L60 L61 L62 L63 L64 | S56 S57 S58 S59 L65 L66 S60 S61 S62 L67 L68 S63 S64 | L70 L71 L72 L73 L74 L75 L76 L77 L78 L79 | L80 L81 L82 L83 | L84 L85 L86 L87 | L88 S69 S70 L89 L90 L91 L92 L93 S71 S72 L94 | L95 S73 S74 S75 S76 L96 L97 L98 S77 S78 S79 L99 L100 L101 L102 L103 S80 S81 S82 S83 S84 L104 L105
sketch "Sketch8" plane through (-0.508, -3.429, 0) normal (-1, 0, 0) x (0, 0, 1)
  line L0 (8.255, 6.858) -> (8.255, 0) projected
  line L1 (8.255, 6.858) -> (0, 6.858) projected
  line L2 (0, 0) -> (6.35, 0)
  line L3 (6.35, 0) -> (6.35, 6.858)
  line L4 (6.35, 6.858) -> (0, 6.858)
  line L5 (0, 6.858) -> (0, 0)
  point P0 (0, 3.429)
  dimension "d80" = 1.905
  constraints: 8 end point, 2 parallel, 1 horizontal, 1 perpendicular, 1 point on line
  measures "d80" distance between parallel lines of L0 L3
extrude "Extrusion9" cut sketch "Sketch8" against normal blind 1.143
body "Solid1"
